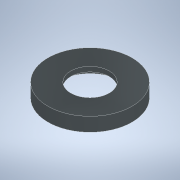
# Autodesk Inventor part: Корпус сальника
Saved by Autodesk Inventor 2021 (Build 250183000, 183)
## iProperties
Created: 2020-11-05
Part Number: Корпус сальника
Material: Чугун, серый
Document SubType Name: Modeling
Designer: Тимоха
Density: 7.15 g/cm^3
Appearance: Чугун серый
Mass: 1505.16 g
Surface Area: 407.904 cm^2
Volume: 210.512 cm^3
Author: Тимоха
Autodesk Inventor part; units mm, degrees
ref_plane "YZ Plane" through (0, 0, 0) normal (1, 0, 0) x (0, 1, 0)
ref_plane "XZ Plane" through (0, 0, 0) normal (0, 1, 0) x (-1, 0, 0)
ref_plane "XY Plane" through (0, 0, 0) normal (0, 0, 1) x (1, 0, 0)
sketch "Эскиз1" plane through (0, 0, 0) normal (0, 0, 1) x (1, 0, 0)
  line L0 (0, 0) -> (0, 20)
  line L1 (69, 0) -> (49, 0)
  line L2 (49, 0) -> (49, 15)
  line L3 (32, 20) -> (32, 15)
  line L4 (32, 15) -> (32, 23)
  line L5 (32, 23) -> (69, 23)
  line L6 (69, 0) -> (69, 23)
  line L7 (32, 15) -> (49, 15)
  dimension "d2" = 20
  dimension "d3" = 15
  dimension "d4" = 32
  dimension "d6" = 8
  dimension "d7" = 17
  constraints: 16 end point, 2 vertical, 1 horizontal, 1 perpendicular, 1 point on line
  measures "d2" distance of L1.start L1.end
  measures "d3" distance of L1.end L2.end
  measures "d4" distance of L0.end L3.start
  measures "d6" distance of L3.end L4.end
  measures "d7" distance of L3.end L2.end
revolve "Вращение1" add sketch "Эскиз1" angle 360 about axis through (0, 0, 0) along (0, 1, 0)
sketch "Эскиз2" plane through (0, 23, 0) normal (0, 1, 0) x (1, 0, 0)
  circle A0 centre (0, 0) radius 32 projected
  circle A1 centre (0, 0) radius 69 projected
  line L0 (0, 0) -> (38.5673, 45.9627)
  line L1 (0, 0) -> (60, 0) construction
  circle A2 centre (38.5673, 45.9627) radius 3
  line L2 (0, 0) -> (-30, 51.9615)
  line L3 (0, 0) -> (60, 0) construction
  circle A3 centre (-30, 51.9615) radius 3
  line L4 (0, 0) -> (-10.4189, -59.0885)
  line L5 (0, 0) -> (60, 0) construction
  circle A4 centre (-10.4189, -59.0885) radius 3
  dimension "d8" = 60
  dimension "d9" = 50
  dimension "d10" = 6
  dimension "d11" = 60
  dimension "d12" = 120
  dimension "d13" = 6
  dimension "d14" = 60
  dimension "d15" = 100
  dimension "d16" = 6
  constraints: 12 end point, 3 centre point, 3 coincident, 3 equal length, 3 horizontal, 1 point on line
  measures "d8" distance of L0.start L0.end
  measures "d9" angle of L1 L0
  measures "d10" diameter of A2
  measures "d11" distance of L0.start L2.end
  measures "d12" angle of L3 L2
  measures "d13" diameter of A3
  measures "d14" distance of L0.start L4.end
  measures "d15" angle of L4 L5
  measures "d16" diameter of A4
extrude "Выдавливание1" cut sketch "Эскиз2" against normal through all contours A2 | A3 | A4
